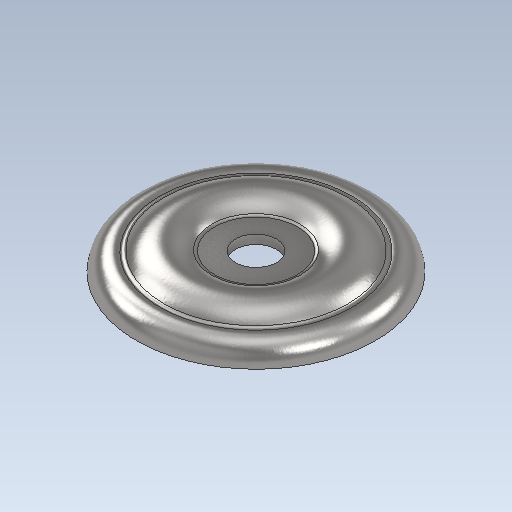
# Autodesk Inventor part: Wheel 75 mm - Part 4
Saved by Autodesk Inventor 2020 (Build 240168000, 168)
## iProperties
Created: 2023-01-26
Part Number: Wheel 75 mm - Part 4
Material: Steel, Galvanized
Document SubType Name: Modeling
Designer: saad.nashed
Density: 7.85 g/cm^3
Appearance: Galvanized
Author: saad.nashed
Autodesk Inventor part; units mm, degrees
ref_plane "YZ Plane" through (0, 0, 0) normal (1, 0, 0) x (0, 1, 0)
ref_plane "XZ Plane" through (0, 0, 0) normal (0, 1, 0) x (-1, 0, 0)
ref_plane "XY Plane" through (0, 0, 0) normal (0, 0, 1) x (1, 0, 0)
sketch "Sketch1" plane through (0, 0, 0) normal (1, 0, 0) x (0, 1, 0)
  line L0 (1.7625, -4) -> (1.7625, -8.0739)
  arc A0 (0.4383, -16.8023) -> (0.5635, -9.7054) centre (-3.8625, -13.1769) ccw
  arc A1 (1.7625, -8.0739) -> (1.9503, -8.6177) centre (2.6438, -8.0739) ccw
  arc A2 (0, -8.0739) -> (0.5635, -9.7054) centre (2.6438, -8.0739) ccw
  arc A3 (-1.7625, -23.2912) -> (1.6153, -18.7582) centre (-1.7625, -19.7662) ccw
  arc A4 (-1.7625, -21.5287) -> (-0.0736, -19.2622) centre (-1.7625, -19.7662) ccw
  arc A5 (1.7859, -17.9382) -> (1.6153, -18.7582) centre (2.4597, -18.5062) ccw
  arc A6 (0.4383, -16.8023) -> (-0.0736, -19.2622) centre (2.4597, -18.5062) ccw
  arc A7 (1.7859, -17.9382) -> (1.9503, -8.6177) centre (-3.8625, -13.1769) ccw
  line L1 (-1.7625, -21.5287) -> (-1.7625, -23.2912)
  line L2 (0, 0) -> (0, 2.3127)
  line L3 (-5.3562, 0) -> (5.0998, 0) projected
  line L4 (1.7625, -4) -> (0, -4)
  line L5 (0, -8.0739) -> (0, -4)
  dimension "d1" = 21.5287
  dimension "d5" = 13.1769
  dimension "d6" = 0.8812
  dimension "d8" = 1.7625
  dimension "d9" = 1.7625
  dimension "d11" = 5.625
  dimension "d12" = 1.7625
  dimension "d13" = 1.7625
  dimension "d14" = 4
  dimension "d15" = 3.525
  constraints: 16 point on circle, 10 end point, 9 tangent, 8 centre point, 3 vertical, 1 concentric, 1 equal radius, 1 horizontal, 1 point on line
  measures "d1" vertical distance of L1.start L2.start
  measures "d5" vertical distance of A0.centre L2.start
  measures "d6" radius of A1
  measures "d8" distance from line of L2 L1.start
  measures "d9" distance between parallel lines of L2 L0
  measures "d11" radius of A0
  measures "d12" radius of A4
  measures "d13" distance of A3.centre L1.start
  measures "d14" distance between parallel lines of L4 L3
  measures "d15" distance edge to line of A7 L5
revolve "Revolution1" add sketch "Sketch1" angle 360 about axis through (0, -10, 0) along (0, 1, 0)
equation "\"d1\" = d2 + 0.3 * d19"
equation "\"d5\" = d32"
equation "\"d6\" = 0.5 * d19"
equation "\"d8\" = d19"
equation "\"d9\" = d3"
equation "\"d11\" = d29"
equation "\"d12\" = d19"
equation "\"d13\" = d12"
equation "\"d14\" = d25"
equation "\"d3\" = d19"
equation "\"d2\" = 21"
equation "\"d19\" = 1.7625"
equation "\"d32\" = 13.176899"
equation "\"d29\" = 5.625"
equation "\"d25\" = 4"
body "Solid1"
